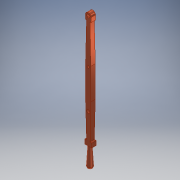
# Autodesk Inventor part: reverse gear rever lever
Saved by Autodesk Inventor 2017 (Build 210142000, 142)
## iProperties
Created: 2018-11-14
Part Number: reverse gear rever lever
Material: Generic
Document SubType Name: Modeling
Designer: User
Density: 1 g/cm^3
Appearance: Default
Author: User
Autodesk Inventor part; units mm, degrees
ref_plane "XZ Plane" through (0, 0, 0) normal (0, 1, 0) x (-1, 0, 0)
ref_plane "XY Plane" through (0, 0, 0) normal (0, 0, 1) x (1, 0, 0)
sketch "Sketch1" plane through (0, 0, 0) normal (0, 1, 0) x (-1, 0, 0)
  line L0 (-3.25, 5) -> (-3.25, 0)
  line L1 (-3.25, 0) -> (3.25, 0)
  line L2 (3.25, 0) -> (3.25, 5)
  line L3 (2, 0) -> (-2, 0)
  line L4 (3, -43) -> (3, -78)
  line L5 (-3, -78) -> (-3, -43)
  line L6 (2, -118) -> (-2, -118)
  circle A0 centre (0, 5) radius 1.75
  arc A1 (3.25, 5) -> (-3.25, 5) centre (0, 5) ccw
  line L7 (2, 0) -> (3, -43)
  line L8 (-3, -43) -> (-2, 0)
  line L9 (3, -78) -> (2, -118)
  line L10 (-2, -118) -> (-3, -78)
  point P0 (0, 0)
  point P1 (0, 0)
  point P2 (0, 0)
  point P3 (0, -43)
  point P4 (0, -78)
  dimension "d0" = 6.5
  dimension "d1" = 5
  dimension "d2" = 6
  dimension "d3" = 4
  dimension "d4" = 3.5
  dimension "d5" = 90
  dimension "d6" = 91.332
  dimension "d7" = 88.568
  dimension "d8" = 91.332
  dimension "d9" = 88.568
  dimension "d10" = 118
  dimension "d11" = 0.25
  dimension "d12" = 6.25
  dimension "d13" = 1.9995
  dimension "d14" = 43
  dimension "d15" = 3.25
  dimension "d16" = 78
  dimension "d17" = 3.25
  dimension "d18" = 0
  dimension "d19" = 3.25
  constraints: 22 end point, 4 parallel, 2 centre point, 2 midpoint, 2 point on circle, 2 tangent, 1 coincident, 1 concentric, 1 horizontal, 1 vertical
  measures "d0" distance of L1.end L0.end
  measures "d1" distance of L0.end L0.start
  measures "d2" distance of L5.start L4.end
  measures "d3" distance of L6.end L6.start
  measures "d4" diameter of A0
  measures "d5" angle of L2 L1
  measures "d6" angle of L7 L3
  measures "d7" angle of L9 L3
  measures "d8" angle of L8 L3
  measures "d9" angle of L10 L3
  measures "d10" distance between parallel lines of L6 L3
  measures "d11" distance between parallel lines of L4 L2
  measures "d12" distance between parallel lines of L5 L2
  measures "d13" distance from line of point (0, 0) L7
  measures "d14" distance from line of point (0, -43) L3
  measures "d15" distance from line of point (0, -43) L2
  measures "d16" distance from line of point (0, -78) L3
  measures "d17" distance from line of point (0, -78) L2
  measures "d18" distance from line of point (0, 0) L3
  measures "d19" distance from line of point (0, 0) L2
extrude "Extrusion1" add sketch "Sketch1" along normal blind 5
sketch "Sketch2" plane through (0, 5, 0) normal (0, 1, 0) x (1, 0, 0)
  circle A0 centre (0, 45) radius 1.25
  circle A1 centre (0, 89) radius 1.75
  circle A2 centre (0, -5) radius 1.75 construction
  circle A3 centre (0, -5) radius 1.75 construction
  point P0 (0, 0)
  point P1 (0, 0)
  dimension "d22" = 2.5
  dimension "d23" = 3.5
  dimension "d24" = 44
  dimension "d25" = 3.5
  dimension "d26" = 50
  dimension "d116" = 45
  dimension "d117" = 0
  constraints: 4 centre point, 2 vertical alignment, 1 coincident, 1 equal radius
  measures "d22" diameter of A0
  measures "d23" diameter of A1
  measures "d24" distance of A1.centre A0.centre
  measures "d25" diameter of A3
  measures "d26" distance of A0.centre A3.centre
  measures "d116" distance of point (0, 0) A0.centre
  measures "d117" distance of point (0, 0) point (0, 0)
extrude "Extrusion2" cut sketch "Sketch2" against normal through all
sketch "Sketch6" plane through (2, 0, -118) normal (0, 0, -1) x (-1, 0, 0)
  line L0 (0, 5) -> (4, 5) projected
  line L1 (0.75, 5) -> (3.25, 5) projected
  line L2 (2, 5) -> (-2, 5)
  line L3 (2, 5) -> (6, 5)
  line L4 (6, 5) -> (6, 0)
  line L5 (6, 0) -> (-2, 0)
  line L6 (5.25, 0) -> (-1.25, 0) projected
  line L7 (-2, 0) -> (-2, 5)
  dimension "d43" = 4
  dimension "d44" = 4
  dimension "d45" = 5
  dimension "d46" = 8
  constraints: 10 end point, 1 collinear, 1 horizontal, 1 midpoint, 1 point on line, 1 vertical
  measures "d43" distance of L2.start L2.end
  measures "d44" distance of L2.start L3.end
  measures "d45" distance of L3.end L4.end
  measures "d46" distance of L4.end L5.end
extrude "Extrusion5" add sketch "Sketch6" along normal blind 5
ref_plane "Work Plane1" through (0, 0, 0) normal (1, 0, 0) x (0, 1, 0)
sketch "Sketch11" plane through (0, 0, 0) normal (1, 0, 0) x (0, 1, 0)
  line L0 (4.51, -121.065) -> (4.51, -116.065) construction
  line L1 (2.01, -122.9844) -> (4.01, -122.9844)
  line L2 (4.01, -122.9844) -> (5.26, -146.065)
  line L3 (5.26, -146.065) -> (2.01, -146.065)
  line L4 (2.01, -146.065) -> (2.01, -122.9844)
  line L5 (0, -118) -> (5, -118) projected
  line L6 (5, -43.75) -> (5, -46.25) projected
  line L7 (5, -87.25) -> (5, -90.75) projected
  line L8 (5, 6.75) -> (5, 3.25) projected
  line L9 (5, 5) -> (5, 5) projected
  line L10 (5, 5) -> (5, 0) projected
  line L11 (5, 0) -> (5, -43) projected
  line L12 (5, -43) -> (5, -78) projected
  line L13 (5, -78) -> (5, -118) projected
  line L14 (5, -118) -> (5, -123) projected
  line L15 (5, -118) -> (5, -123) projected
  line L16 (5, -118) -> (5, -78) projected
  line L17 (5, -78) -> (5, -43) projected
  line L18 (5, -43) -> (5, 0) projected
  line L19 (5, 0) -> (5, 5) projected
  line L20 (0.51, -143.3532) -> (0.51, -134.9626)
  line L21 (4.635, -134.5247) -> (4.635, -134.5247)
  line L22 (7.1466, -143.3532) -> (7.1466, -134.9626)
  point P0 (0, 0)
  point P1 (0, 0)
  dimension "d67" = 2
  dimension "d68" = 3.25
  dimension "d72" = 2.6467
  dimension "d73" = 30
  dimension "d76" = 2.6467
  dimension "d78" = 1.5
  dimension "d80" = 177.138
  dimension "d81" = 6.6366
  dimension "d82" = 3.1
  dimension "d107" = 0.49
  dimension "d109" = 16.9626
  dimension "d110" = 25.3532
  dimension "d111" = 3.065
  dimension "d112" = 16.9626
  dimension "d113" = 25.3532
  dimension "d114" = 7.1466
  constraints: 16 end point, 3 vertical, 2 midpoint, 2 parallel, 1 horizontal
  measures "d67" distance of L1.start L1.end
  measures "d68" distance of L2.end L3.end
  measures "d72" distance from line of point (0, 0) L2
  measures "d73" distance from line of L0.end L3
  measures "d76" distance from line of point (0, 0) L2
  measures "d78" distance between parallel lines of L4 L20
  measures "d80" angle of L20 L21
  measures "d81" distance between parallel lines of L20 L22
  measures "d82" angle of L2 L22
  measures "d107" distance between parallel lines of L6 L0
  measures "d109" distance from line of L22.end L5
  measures "d110" distance from line of L22.start L5
  measures "d111" distance from line of L0.start L5
  measures "d112" distance from line of L20.end L5
  measures "d113" distance from line of L20.start L5
  measures "d114" distance from line of point (0, 0) L22
revolve "Revolution2" add sketch "Sketch11" angle 360 about axis through (0, 2.01, -146.065) along (0, 0, 1)
fillet "Fillet1" radius 3 1 edges at (0, -1.24, -146.065)
body "Solid1"
